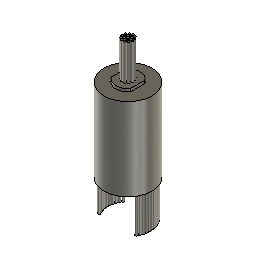
single_axis_test_jig (Autodesk Fusion 360 archive; units mm, degrees)
design "slip_ring_6.75Rx23.2Lmm"
Autodesk Fusion 360 part; units mm, degrees
note: some values were not read from the file. Set by a fixed rule: which sketch regions a step uses.
(part 1 of 4)
sketch "Sketch1" plane through (0, 0, 0) normal (0, 0, 1) x (1, 0, 0)
sketch "Sketch2" plane through (0, 0, 0) normal (0, 0, 1) x (1, 0, 0)
  circle A0 centre (0, 0) radius 6.75
  dimension "d1" = 13.5
  constraint coincident A0.centre origin
  measures "d1" diameter of A0
extrude "Extrude1" add sketch "Sketch2" along normal blind 23.2
sketch "Sketch3" plane through (0, 0, 23.2) normal (0, 0, 1) x (-1, 0, 0)
  circle A0 centre (0, 0) radius 6.75
  line L0 (-2.75, -1.9994) -> (-2.75, 1.9994)
  line L1 (2.75, 1.9994) -> (2.75, -1.9994)
  arc A1 (2.75, 1.9994) -> (-2.75, 1.9994) centre (0, 0) ccw
  arc A2 (-2.75, -1.9994) -> (2.75, -1.9994) centre (0, 0) ccw
  dimension "d4" = 6.8
  constraint coincident A0.centre A1.centre
  constraint vertical L0
  constraint vertical L1
  constraint concentric A1 A2
  measures "d4" diameter of A1
extrude "Extrude2" add sketch "Sketch3" along normal blind 0.8 contours L0 L1 A1 A2
sketch "Sketch5" plane through (0, 0, 24) normal (0, 0, 1) x (-1, 0, 0)
  arc A0 (2.75, 1.9994) -> (-2.75, 1.9994) centre (0, 0) ccw
  line L0 (-2.75, 1.9994) -> (-2.75, -1.9994)
  arc A1 (-2.75, -1.9994) -> (2.75, -1.9994) centre (0, 0) ccw
  line L1 (2.75, -1.9994) -> (2.75, 1.9994)
  circle A2 centre (0, 0) radius 0.3
  circle A3 centre (0, -0.7865) radius 0.3
  circle A4 centre (0.5561, -0.5561) radius 0.3
  circle A5 centre (0.7865, 0) radius 0.3
  circle A6 centre (0.5561, 0.5561) radius 0.3
  circle A7 centre (0, 0.7865) radius 0.3
  circle A8 centre (-0.5561, 0.5561) radius 0.3
  circle A9 centre (-0.7865, 0) radius 0.3
  circle A10 centre (-0.5561, -0.5561) radius 0.3
  circle A11 centre (0.007, -1.4) radius 0.3
  circle A12 centre (0.7628, -1.174) radius 0.3
  circle A13 centre (1.2764, -0.5752) radius 0.3
  circle A14 centre (1.3848, 0.2061) radius 0.3
  circle A15 centre (1.0535, 0.9221) radius 0.3
  circle A16 centre (0.3877, 1.3453) radius 0.3
  circle A17 centre (-0.4011, 1.3413) radius 0.3
  circle A18 centre (-1.0626, 0.9115) radius 0.3
  circle A19 centre (-1.3867, 0.1923) radius 0.3
  circle A20 centre (-1.2706, -0.5879) radius 0.3
  circle A21 centre (-0.751, -1.1815) radius 0.3
  dimension "d18" = 0.6
  dimension "d19" = 0.6
  dimension "d21" = 360
  dimension "d22" = 0.6
  dimension "d23" = 0.7865
  dimension "d24" = 1.4
  dimension "d26" = 360
  constraint coincident A0.centre A1.centre
  measures "d18" diameter of A2
  measures "d19" diameter of A3
  measures "d22" diameter of A11
  measures "d23" distance of A0.centre A3.centre
  measures "d24" vertical distance of A0.centre A11.centre
extrude "Extrude4" add sketch "Sketch5" along normal blind 10 contours A2 | A3 | A4 | A10 | A5 | A9 | A6 | A8 | A7 | A11 | A12 | A13 | A14 | A15 | A16 | A17 | A18 | A19 | A20 | A21
sketch "Sketch6" plane through (0, 0, 0) normal (0, 0, -1) x (1, 0, 0)
  circle A0 centre (0, 0) radius 6.75
  circle A1 centre (0, 0) radius 5.25
  circle A2 centre (0, 0) radius 6 construction
  circle A3 centre (-6, 0) radius 0.35
  circle A4 centre (-5.9527, -0.752) radius 0.35
  circle A5 centre (-5.8115, -1.4921) radius 0.35
  circle A6 centre (-5.5787, -2.2087) radius 0.35
  circle A7 centre (-5.2578, -2.8905) radius 0.35
  circle A8 centre (-4.8541, -3.5267) radius 0.35
  circle A9 centre (4.8541, -3.5267) radius 0.35
  circle A10 centre (5.2578, -2.8905) radius 0.35
  circle A11 centre (5.5787, -2.2087) radius 0.35
  circle A12 centre (5.8115, -1.4921) radius 0.35
  circle A13 centre (5.9527, -0.752) radius 0.35
  circle A14 centre (6, 0) radius 0.35
  circle A15 centre (5.9527, 0.752) radius 0.35
  circle A16 centre (5.8115, 1.4921) radius 0.35
  circle A17 centre (5.5787, 2.2087) radius 0.35
  circle A18 centre (5.2578, 2.8905) radius 0.35
  circle A19 centre (-5.2578, 2.8905) radius 0.35
  circle A20 centre (-5.5787, 2.2087) radius 0.35
  circle A21 centre (-5.8115, 1.4921) radius 0.35
  circle A22 centre (-5.9527, 0.752) radius 0.35
  dimension "d29" = 10.5
  dimension "d30" = 12
  dimension "d31" = 0.7
  dimension "d33" = 360
  constraint concentric A0 A1
  constraint concentric A1 A2
  constraint coincident A2 A3.centre
  measures "d29" diameter of A1
  measures "d30" diameter of A2
  measures "d31" diameter of A3
extrude "Extrude5" add sketch "Sketch6" along normal blind 10 contours A3 | A4 | A5 | A6 | A7 | A8 | A9 | A10 | A11 | A12 | A13 | A14 | A15 | A16 | A17 | A18 | A19 | A20 | A21 | A22

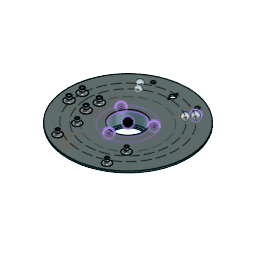
design "top_plate"
Autodesk Fusion 360 part; units mm, degrees
sketch "Sketch1" plane through (0, 0, 0) normal (0, 0, 1) x (1, 0, 0)
  circle A0 centre (0, 0) radius 80
  dimension "d1" = 160
  constraint coincident A0.centre origin
  measures "d1" diameter of A0
extrude "Extrude1" add sketch "Sketch1" along normal blind 2
sketch "Sketch4" plane through (0, 0, 2) normal (0, 0, 1) x (-1, 0, 0)
  circle A0 centre (0, 0) radius 80
  circle A1 centre (0, 0) radius 18
  dimension "d9" = 36
  constraint concentric A0 A1
  measures "d9" diameter of A1
extrude "Extrude3" cut sketch "Sketch4" against normal blind 20 contours A1
sketch "Sketch5" plane through (0, 0, 2) normal (0, 0, 1) x (-1, 0, 0)
  circle A0 centre (0, 0) radius 18
  circle A1 centre (0, 0) radius 80
  circle A2 centre (0, 0) radius 21
  circle A3 centre (0, 0) radius 30
  dimension "d12" = 42
  dimension "d13" = 60
  constraint coincident A0.centre A1.centre
  constraint concentric A2 A3
  measures "d12" diameter of A2
  measures "d13" diameter of A3
extrude "Extrude4" add sketch "Sketch5" against normal blind 19 contours A3
sketch "Sketch6" plane through (0, 0, 2) normal (0, 0, -1) x (-1, 0, 0)
  circle A0 centre (0, 0) radius 21
  circle A1 centre (0, 0) radius 28
  circle A2 centre (0, -25.5) radius 1.6
  circle A3 centre (0, 0) radius 80
  circle A4 centre (0, 0) radius 18
  dimension "d118" = 3.2
  dimension "d119" = 25.5
  constraint vertical A0.centre A2.centre
  measures "d118" diameter of A2
  measures "d119" distance of A0.centre A2.centre
extrude "Extrude5" cut sketch "Sketch6" along normal blind 6.3 contours A2
pattern_circular "C-Pattern2" count 3 over 360 about axis through (0, 0, 2) along (0, 0, -1) of "Extrude5"
sketch "Sketch7" plane through (0, 0, 0) normal (0, 0, -1) x (1, 0, 0)
  circle A0 centre (0, 0) radius 18
  circle A1 centre (0, 0) radius 80
  circle A2 centre (0, 0) radius 45 construction
  circle A3 centre (0, 0) radius 21
  circle A4 centre (0, 0) radius 30
  dimension "d21" = 90
  constraint concentric A0 A2
  measures "d21" diameter of A2
sketch "Sketch8" plane through (0, 0, 0) normal (0, 0, -1) x (1, 0, 0)
  circle A0 centre (0, -60) radius 3.5
  circle A1 centre (0, -65.5) radius 1
  circle A2 centre (0, -54.5) radius 1
  dimension "d22" = 7
  dimension "d23" = 2
  dimension "d24" = 2
  measures "d22" diameter of A0
  measures "d23" diameter of A1
  measures "d24" diameter of A2
extrude "Extrude6" cut sketch "Sketch8" against normal blind 2
move_face "OffsetFaces1" offset -0.2 1 faces at (20.8956, -2.0909, -11.3333)
ref_plane "WorkPlane1" through (0, 0, 12.125) normal (-0.819152, 0.573576, 0) x (0, 0, 1)
ref_plane "WorkPlane2" through (0, 0, 12.125) normal (-0.819152, -0.573576, 0) x (0, 0, 1)
sketch "Sketch9" plane through (0, 0, 2) normal (0, 0, 1) x (-1, 0, 0)
  circle A0 centre (0, 0) radius 80
  circle A1 centre (0, 0) radius 55 construction
  circle A2 centre (0, 0) radius 64.5 construction
  circle A3 centre (-22.0836, -12.75) radius 1.6
  circle A4 centre (22.0836, -12.75) radius 1.6
  circle A5 centre (0, 25.5) radius 1.6
  dimension "d31" = 110
  dimension "d32" = 129
  constraint coincident A0.centre A1.centre
  constraint concentric A0 A2
  measures "d31" diameter of A1
  measures "d32" diameter of A2
sketch "Sketch10" plane through (0, 0, 0) normal (-0.819152, -0.573576, 0) x (0, 0, 1)
  line L0 (2, 55) -> (2, 64.5) construction
  line L1 (2, 64.5) -> (2, 65)
  dimension "d34" = 9.5
  dimension "d43" = 0.5
  constraint vertical L0
  constraint parallel L0 L1
  measures "d34" distance of L0.start L0.end
  measures "d43" distance of L0.end L1.end
sketch "Sketch11" plane through (0, 0, 0) normal (-0.819152, 0.573576, 0) x (0, 0, 1)
  line L0 (2, 55) -> (2, 64.5) construction
  line L1 (2, 64.5) -> (2, 65) construction
  dimension "d36" = 9.5
  constraint vertical L0
  constraint parallel L0 L1
  measures "d36" distance of L0.start L0.end
sketch "Sketch12" plane through (0, 0, 2) normal (0, 0, 1) x (-1, 0, 0)
  circle A0 centre (-36.9957, -52.8353) radius 1.25
  circle A1 centre (-31.5467, -45.0534) radius 1.25
  circle A2 centre (31.5467, -45.0534) radius 1.25
  circle A3 centre (36.9957, -52.8353) radius 1.25
  point P0 (-36.9957, -52.8353)
  point P1 (-31.5467, -45.0534)
  point P2 (31.5467, -45.0534)
  point P3 (36.9957, -52.8353)
  dimension "d37" = 2.5
  dimension "d38" = 2.5
  dimension "d39" = 2.5
  dimension "d40" = 2.5
  constraint coincident P0 A0.centre
  constraint coincident P1 A1.centre
  constraint coincident P2 A2.centre
  constraint coincident P3 A3.centre
  measures "d37" diameter of A0
  measures "d38" diameter of A1
  measures "d39" diameter of A2
  measures "d40" diameter of A3
extrude "Extrude7" cut sketch "Sketch12" against normal blind 2
sketch "Sketch13" plane through (0, 0, 2) normal (0, 0, 1) x (-1, 0, 0)
  circle A0 centre (37.2825, -53.2449) radius 1.25
  point P0 (37.2825, -53.2449)
  dimension "d44" = 2.5
  constraint coincident P0 A0.centre
  measures "d44" diameter of A0
sketch "Sketch14" plane through (0, 0, 2) normal (0, 0, 1) x (-1, 0, 0)
  point P0 (-37.2825, -53.2449)
sketch "Sketch15" plane through (0, 0, 2) normal (0, 0, 1) x (-1, 0, 0)
  line L0 (-38.0196, -52.1183) -> (-38.3064, -52.5279)
  circle A0 centre (-37.2825, -53.2449) radius 1.25
  circle A1 centre (-36.9957, -52.8353) radius 1.25
  line L1 (-35.9717, -53.5523) -> (-36.2585, -53.9619)
  circle A2 centre (-31.5467, -45.0534) radius 1.25
  circle A3 centre (31.5467, -45.0534) radius 1.25
  circle A4 centre (-36.9957, -52.8353) radius 1.25
  circle A5 centre (36.9957, -52.8353) radius 1.25
  circle A6 centre (0, -60) radius 3.5
  circle A7 centre (0, -65.5) radius 1
  circle A8 centre (0, -54.5) radius 1
  circle A9 centre (0, 0) radius 80
  circle A10 centre (0, 0) radius 18
  circle A11 centre (-22.0836, -12.75) radius 1.6
  circle A12 centre (22.0836, -12.75) radius 1.6
  circle A13 centre (0, 25.5) radius 1.6
  point P0 (-36.9957, -52.8353)
  constraint tangent L0 A0
  constraint coincident L0.end A0
  constraint coincident L0.start A1
  constraint tangent A1 L1
  constraint coincident A1 L1.start
  constraint coincident A0 L1.end
  constraint coincident P0 A1.centre
extrude "Extrude8" cut sketch "Sketch15" against normal blind 2 contours L0 A0 A1 A4 | A0 A1 A4 | A0 A1 L1 A4 picked at (-38.0226, -54.0336)
sketch "Sketch16" plane through (0, 0, 2) normal (0, 0, 1) x (-1, 0, 0)
  line L0 (36.2585, -53.9619) -> (35.9717, -53.5523)
  line L1 (31.5467, -45.0534) -> (36.9957, -52.8353)
  circle A0 centre (37.2825, -53.2449) radius 1.25
  circle A1 centre (36.9957, -52.8353) radius 1.25
  line L2 (38.3064, -52.5279) -> (38.0196, -52.1183)
  constraint parallel L0 L1
  constraint tangent L0 A0
  constraint coincident L0.start A0
  constraint coincident L0.end A1
  constraint parallel L1 L2
  constraint tangent A1 L2
  constraint coincident A1 L2.end
  constraint coincident A0 L2.start
extrude "Extrude9" cut sketch "Sketch16" sketch "Sketch13" against normal blind 2 contours L0 A0 A1 | A0 A1 L2 of sketch 2
move_face "OffsetFaces3" offset 0.4 1 faces at (21.0947, -2.1108, -5.6667)
move_face "OffsetFaces4" offset -0.3 1 faces at (4.8751, -17.3272, 0.6667)
move_face "OffsetFaces5" offset -0.2 1 faces at (3.4826, 60.3485, 0.6667)
move_face "OffsetFaces8" offset -0.15 10 faces at (-32.6985, 44.5678, 0.6667) (-37.0808, 54.4785, 0.6667) (-36.0673, 53.6888, 0.6667) (-35.9054, 53.4468, 0.6667) (-38.1152, 52.2549, 0.6667) (32.2249, 46.1034, 0.6667) (37.9826, 52.0682, 0.6667) (36.1629, 53.8253, 0.6667) (38.3727, 52.6334, 0.6667) (38.2108, 52.3914, 0.6667)
move_face "OffsetFaces9" offset -0.15 2 faces at (-0.9215, 54.8884, 1.3333) (-0.9802, 65.3019, 1.3333)
sketch "Sketch17" plane through (0, 0, 2) normal (0, 0, 1) x (-1, 0, 0)
  line L0 (0, 35) -> (0, 61.15) construction
  line L1 (0, 35) -> (-33.075, 35) construction
  line L2 (0, 35) -> (33.075, 35) construction
  line L3 (0, 61.15) -> (-33.075, 61.15) construction
  line L4 (0, 61.15) -> (33.075, 61.15) construction
  circle A0 centre (33.075, 35) radius 2.5
  circle A1 centre (-33.075, 35) radius 2.5
  circle A2 centre (33.075, 61.15) radius 2.5
  circle A3 centre (-33.075, 61.15) radius 2.5
  dimension "d59" = 26.15
  dimension "d60" = 33.075
  dimension "d61" = 33.075
  dimension "d62" = 33.075
  dimension "d63" = 33.075
  dimension "d64" = 5
  dimension "d65" = 5
  dimension "d66" = 5
  dimension "d67" = 5
  constraint vertical L0
  constraint perpendicular L0 L1
  constraint perpendicular L0 L2
  constraint perpendicular L0 L3
  constraint perpendicular L0 L4
  constraint coincident L2.end A0.centre
  constraint coincident L1.end A1.centre
  constraint coincident L4.end A2.centre
  constraint coincident L3.end A3.centre
  measures "d59" distance of L0.start L0.end
  measures "d60" distance of L0.start L1.end
  measures "d61" distance of L0.start L2.end
  measures "d62" distance of L0.end L3.end
  measures "d63" distance of L0.end L4.end
  measures "d64" diameter of A0
  measures "d65" diameter of A1
  measures "d66" diameter of A2
  measures "d67" diameter of A3
extrude "Extrude11" add sketch "Sketch17" along normal blind 6
fillet "Fillet1" radius 3 4 edges at (-30.7442, -62.054, 2) (-30.7442, -35.904, 2) (35.4058, -35.904, 2) (35.4058, -62.054, 2)
sketch "Sketch18" plane through (0, 0, 8) normal (0, 0, 1) x (-1, 0, 0)
  circle A0 centre (33.075, 35) radius 2.5
  circle A1 centre (33.075, 35) radius 1.55
  dimension "d73" = 3.1
  constraint concentric A0 A1
  measures "d73" diameter of A1
sketch "Sketch19" plane through (0, 0, 8) normal (0, 0, 1) x (-1, 0, 0)
  circle A0 centre (33.075, 61.15) radius 2.5
  circle A1 centre (33.075, 61.15) radius 1.55
  dimension "d74" = 3.1
  constraint concentric A0 A1
  measures "d74" diameter of A1
sketch "Sketch20" plane through (0, 0, 8) normal (0, 0, 1) x (-1, 0, 0)
  circle A0 centre (-33.075, 61.15) radius 2.5
  circle A1 centre (-33.075, 61.15) radius 1.55
  dimension "d75" = 3.1
  constraint concentric A0 A1
  measures "d75" diameter of A1
sketch "Sketch21" plane through (0, 0, 8) normal (0, 0, 1) x (-1, 0, 0)
  circle A0 centre (-33.075, 35) radius 2.5
  circle A1 centre (-33.075, 35) radius 1.55
  dimension "d76" = 3.1
  constraint concentric A0 A1
  measures "d76" diameter of A1
extrude "Extrude12" cut sketch "Sketch20" sketch "Sketch19" sketch "Sketch18" sketch "Sketch21" against normal blind 5 contours A1 of sketch 2 contours A1 of sketch 3 contours A1 of sketch 4 contours A1
sketch "Sketch22" plane through (0, 0, 2) normal (0, 0, 1) x (-1, 0, 0)
  line L0 (42, 0) -> (64.86, 0) construction
  line L1 (42, 0) -> (42, 14.113) construction
  line L2 (64.86, 0) -> (64.86, 14.113) construction
  line L3 (42, 0) -> (42, -3.667) construction
  line L4 (64.86, 0) -> (64.86, -3.667) construction
  circle A0 centre (64.86, -3.667) radius 3
  circle A1 centre (64.86, 14.113) radius 3
  circle A2 centre (42, -3.667) radius 3
  circle A3 centre (42, 14.113) radius 3
  dimension "d79" = 22.86
  dimension "d80" = 14.113
  dimension "d81" = 14.113
  dimension "d82" = 3.667
  dimension "d83" = 3.667
  dimension "d84" = 6
  dimension "d85" = 6
  dimension "d86" = 6
  dimension "d87" = 6
  constraint horizontal L0
  constraint perpendicular L0 L1
  constraint perpendicular L0 L2
  constraint perpendicular L0 L3
  constraint perpendicular L0 L4
  constraint coincident L4.end A0.centre
  constraint coincident L2.end A1.centre
  constraint coincident L3.end A2.centre
  constraint coincident L1.end A3.centre
  measures "d79" distance of L0.start L0.end
  measures "d80" distance of L0.start L1.end
  measures "d81" distance of L0.end L2.end
  measures "d82" distance of L0.start L3.end
  measures "d83" distance of L0.end L4.end
  measures "d84" diameter of A0
  measures "d85" diameter of A1
  measures "d86" diameter of A2
  measures "d87" diameter of A3
extrude "Extrude13" add sketch "Sketch22" along normal blind 6
fillet "Fillet2" radius 3 4 edges at (-62.063, -15.1978, 2) (-39.203, -15.1978, 2) (-39.203, 2.5822, 2) (-62.063, 2.5822, 2)
sketch "Sketch23" plane through (0, 0, 8) normal (0, 0, 1) x (-1, 0, 0)
  circle A0 centre (42, -3.667) radius 3
  circle A1 centre (42, -3.667) radius 2.2
  dimension "d92" = 4.4
  constraint concentric A0 A1
  measures "d92" diameter of A1
sketch "Sketch24" plane through (0, 0, 8) normal (0, 0, 1) x (-1, 0, 0)
  circle A0 centre (42, 14.113) radius 3
  circle A1 centre (42, 14.113) radius 2.2
  dimension "d93" = 4.4
  constraint concentric A0 A1
  measures "d93" diameter of A1
sketch "Sketch25" plane through (0, 0, 8) normal (0, 0, 1) x (-1, 0, 0)
  circle A0 centre (64.86, 14.113) radius 3
  circle A1 centre (64.86, 14.113) radius 2.2
  dimension "d94" = 4.4
  constraint concentric A0 A1
  measures "d94" diameter of A1
sketch "Sketch26" plane through (0, 0, 8) normal (0, 0, 1) x (-1, 0, 0)
  circle A0 centre (64.86, -3.667) radius 3
  circle A1 centre (64.86, -3.667) radius 2.2
  dimension "d95" = 4.4
  constraint concentric A0 A1
  measures "d95" diameter of A1
extrude "Extrude14" cut sketch "Sketch26" sketch "Sketch25" sketch "Sketch24" sketch "Sketch23" against normal blind 5 contours A1 of sketch 2 contours A1 of sketch 3 contours A1 of sketch 4 contours A1
sketch "Sketch27" plane through (0, 0, -17) normal (0, 0, -1) x (1, 0, 0)
  circle A0 centre (0, 0) radius 20.8
  circle A1 centre (0, 0) radius 30
  circle A2 centre (0, -24.5) radius 2.2
  circle A3 centre (-21.2176, 12.25) radius 2.2
  circle A4 centre (21.2176, 12.25) radius 2.2
sketch "Sketch28" plane through (0, 0, -17) normal (0, 0, -1) x (1, 0, 0)
  circle A0 centre (0, 0) radius 20.8
  circle A1 centre (0, 0) radius 30
  circle A2 centre (-0.3894, 0) radius 18
  dimension "d103" = 36
  measures "d103" diameter of A2
extrude "Extrude16" add sketch "Sketch28" against normal blind 2 contours A0
sketch "Sketch29" plane through (0, 0, 2) normal (0, 0, 1) x (-1, 0, 0)
sketch "Sketch30" plane through (0, 0, 2) normal (0, 0, 1) x (-1, 0, 0)
  circle A0 centre (0, 0) radius 21.075
  dimension "d106" = 42.15
  constraint coincident A0.centre origin
  measures "d106" diameter of A0
extrude "Extrude17" cut sketch "Sketch30" against normal blind 17
sketch "Sketch31" plane through (0, 0, 2) normal (0, 0, 1) x (-1, 0, 0)
  circle A0 centre (0, 0) radius 70 construction
  circle A1 centre (29.7262, -63.3747) radius 2.6
  circle A2 centre (-29.7262, -63.3747) radius 2.6
  line L0 (31.5467, -45.0534) -> (36.9957, -52.8353)
  line L1 (-31.5467, -45.0534) -> (-36.9957, -52.8353)
  dimension "d109" = 5.2
  dimension "d110" = 5.2
  dimension "d111" = 12
  dimension "d112" = 12
  dimension "d115" = 140
  constraint coincident A0.centre origin
  constraint coincident A0 A1.centre
  constraint coincident A0 A2.centre
  measures "d109" diameter of A1
  measures "d110" diameter of A2
  measures "d111" distance of A1.centre L0
  measures "d112" distance of A2.centre L1
  measures "d115" diameter of A0
extrude "Extrude18" cut sketch "Sketch31" against normal blind 3
sketch "Sketch32" plane through (0, 0, -17) normal (0, 0, -1) x (1, 0, 0)
  circle A0 centre (0, 0) radius 30
  circle A1 centre (0, 0) radius 18
  circle A2 centre (-0.3894, 0) radius 18
  dimension "d120" = 36
  measures "d120" diameter of A1
chamfer "Chamfer1" distance 0.2 angle 45 4 edges at (34.5201, -35.5605, 8) (34.5201, -61.7105, 8) (-31.6299, -61.7105, 8) (-31.6299, -35.5605, 8)
chamfer "Chamfer1" distance 0.2 angle 45 4 edges at (-39.9489, -14.9086, 8) (-39.9489, 2.8714, 8) (-62.8089, 2.8714, 8) (-62.8089, -14.9086, 8)
equation "d119 = ( 51 / 2 ) * 1 mm"

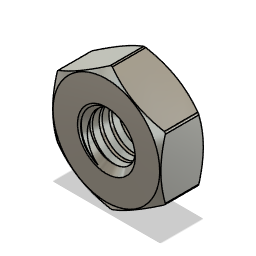
design "M2.5x2mm_hex_nut"
Autodesk Fusion 360 part; units mm, degrees
sketch "Skizze1" plane through (0, 0, 0) normal (0, 0, 1) x (1, 0, 0)
  line L0 (-2.5, -1.4434) -> (0, -2.8868)
  line L1 (0, -2.8868) -> (2.5, -1.4434)
  line L2 (2.5, -1.4434) -> (2.5, 1.4434)
  line L3 (2.5, 1.4434) -> (0, 2.8868)
  line L4 (0, 2.8868) -> (-2.5, 1.4434)
  line L5 (-2.5, 1.4434) -> (-2.5, -1.4434)
  dimension "d3" = 2.5
  constraint vertical L5
  measures "d3" distance of origin L5
extrude "Extrusion1" add sketch "Skizze1" along normal mid plane 2
sketch "Skizze2" plane through (0, 0, 1) normal (0, 0, 1) x (1, 0, 0)
  line L0 (-2.5, 1.4434) -> (-2.5, -1.4434)
  line L1 (-2.5, -1.4434) -> (0, -2.8868)
  line L2 (0, -2.8868) -> (2.5, -1.4434)
  line L3 (2.5, -1.4434) -> (2.5, 1.4434)
  line L4 (2.5, 1.4434) -> (0, 2.8868)
  line L5 (0, 2.8868) -> (-2.5, 1.4434)
hole "Bohrung1" at (0, 0, 1) direction (0, 0, -1) diameter 2.076 end through all
thread "Gewinde1" "ISO Metric profile 2.5 M2.5x0.45 6H" major diameter 2.58 minor diameter 2.0755 pitch 0.45 angle 60 modelled right hand crest width 0.1211 on face at (0.1034, -1.0328, -0.3333) crest through (1.0377, 0, 0.8875)
sketch "Skizze4" plane through (0, 0, 0) normal (1, 0, 0) x (0, 0, -1)
  line L0 (1, 1.4434) -> (1, 2.8868)
  line L1 (1, -2.8868) -> (1, -1.4434)
  line L2 (1, 2.8868) -> (-1, 2.8868)
  line L3 (0.7575, 2.8868) -> (1, 2.4668)
  line L4 (1, 2.8868) -> (0.8181, 2.7818) construction
  line L5 (1, 2.4668) -> (1, 0)
  line L6 (0.7575, 2.8868) -> (0, 2.8868)
  line L7 (0, 1.75) -> (0, 22.5) construction
  line L8 (-0.7575, 2.8868) -> (0, 2.8868)
  line L9 (-0.7575, 2.8868) -> (-1, 2.4668)
  line L10 (-1, 2.4668) -> (-1, 0)
  line L11 (-1, 0) -> (1, 0)
  line L12 (-1, 3.3068) -> (0, 3.3068)
  line L13 (1, 3.3068) -> (0, 3.3068)
  line L14 (1, 3.3068) -> (1.42, 2.5793)
  line L15 (1.42, 2.5793) -> (1.42, -0.42)
  line L16 (-1.42, -0.42) -> (1.42, -0.42)
  line L17 (-1.42, 2.5793) -> (-1.42, -0.42)
  line L18 (-1, 3.3068) -> (-1.42, 2.5793)
  line L19 (-1, 0) -> (-1.42, 0)
  line L20 (1, 0) -> (1.42, 0)
  line L21 (1, -1.4434) -> (1, 1.4434)
  line L22 (-1.75, 0) -> (-22.5, 0)
  dimension "d18" = 0.21
  dimension "d19" = 0.42
  dimension "d23" = 150
  constraint coincident L2 L3.start
  constraint coincident L0 L3.end
  constraint coincident L0.end L2.start
  constraint midpoint L2 L6.end
  constraint symmetric L3.start L7 L8.start
  constraint symmetric L3.end L7 L9.end
  constraint symmetric L5.end L7 L10.end
  constraint symmetric L6.end L7 L8.end
  constraint coincident L17 L19.end
  constraint perpendicular L17 L19
  constraint coincident L15 L20.end
  constraint perpendicular L15 L20
  constraint perpendicular L3 L4
  constraint coincident L3 L4.end
  constraint vertical L10
  constraint collinear L19 L22
  measures "d18" distance of L0.end L4.end
  measures "d23" angle of L3 L5
revolve "Drehen1" cut sketch "Skizze4" angle 360 about axis through (0, 0, 1.75) along (0, 0, 1) contours L0 L2 L5 L6 L8 L9 L10 L12 L13 L14 L15 L17 L18 L19 L20 L21 | L0 L2 L3
fillet "Abrundung1" radius 0.1 6 edges at (2.5, 1.4434, 0) (2.5, -1.4434, 0) (0, -2.8868, 0) (-2.5, -1.4434, 0) (0, 2.8868, 0) (-2.5, 1.4434, 0)
sketch "Skizze5" plane through (0, 0, 0) normal (1, 0, 0) x (0, 0, -1)
  line L0 (-1, 1.3328) -> (-0.7172, 1.05)
  line L1 (-0.7172, 1.05) -> (0, 1.05)
  line L2 (0, 1.75) -> (0, 22.5)
  line L3 (0, 1.05) -> (0, 0) construction
  line L4 (-0.7172, 1.05) -> (-1, 1.05) construction
  line L5 (-1, 1.05) -> (-0.8586, 1.1914) construction
  line L6 (-1, 1.3328) -> (-1, 0)
  line L7 (-1, 0) -> (0, 0)
  line L8 (0.7172, 1.05) -> (0, 1.05)
  line L9 (1, 1.3328) -> (0.7172, 1.05)
  line L10 (1, 1.3328) -> (1, 0)
  line L11 (1, 0) -> (0, 0)
  line L12 (-1, 2.4668) -> (-1, -2.4668)
  dimension "d28" = 1.05
  dimension "d29" = 0.2
  dimension "d31" = 45
  constraint horizontal L1
  constraint coincident L1.end L2
  constraint coincident L3.end L7.end
  constraint coincident L0 L5.end
  constraint perpendicular L0 L5
  constraint symmetric L0.start L2 L9.start
  constraint symmetric L0.end L2 L8.start
  constraint symmetric L1.end L2 L3.start
  constraint symmetric L2 L6.end L10.end
  constraint symmetric L2 L3.end L7.end
  constraint horizontal L7
  constraint vertical L6
  constraint horizontal L4
  constraint coincident L4.end L6
  constraint collinear L6 L12
  measures "d28" distance of L1.end L3.end
  measures "d29" distance of L4.end L5.end
  measures "d31" angle of L0 L6
revolve "Drehen2" cut sketch "Skizze5" angle 360 about axis through (0, 0, 1.75) along (0, 0, 1)
equation "HexWidth = 5 mm" comment "Side-to-side width"
equation "Height = 2 mm"
equation "d3 = HexWidth / 2"
equation "d4 = Height"
equation "ChamferDepth = 0.21 mm" comment "Corner chamfer depth"
equation "ChamferAngle = 30 deg" comment "Corner chamfer angle"
equation "ThreadChamferDepth = 0.2 mm"
equation "d18 = ChamferDepth"
equation "d19 = 2 * ChamferDepth"
equation "SideFillet = 0.1 mm" comment "Fillet of the sides"
equation "d22 = SideFillet"
equation "d23 = 180 deg - ChamferAngle"
equation "ThreadChamferAngle = 45 deg"
equation "CoreDrill = 2.1 mm" comment "Core drill size for the given thread. Used to compute the thread chamfer."
equation "d28 = CoreDrill / 2"
equation "d29 = ThreadChamferDepth"
equation "d31 = ThreadChamferAngle"
named bodies: "Nut"

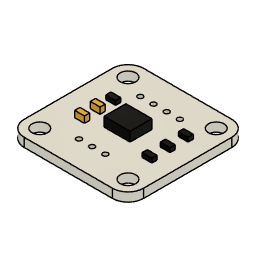
design "AS5600"
Autodesk Fusion 360 part; units mm, degrees
sketch "Sketch2" plane through (0, 0, 0) normal (0, 1, 0) x (1, 0, 0)
  line L0 (-8.5, -11.5) -> (8.5, -11.5)
  line L1 (11.5, -8.5) -> (11.5, 8.5)
  line L2 (8.5, 11.5) -> (-8.5, 11.5)
  line L3 (-11.5, 8.5) -> (-11.5, -8.5)
  line L4 (-11.5, -11.5) -> (11.5, 11.5) construction
  line L5 (11.5, -11.5) -> (-11.5, 11.5) construction
  line L6 (-8.5, 8.5) -> (8.5, 8.5) construction
  line L7 (8.5, 8.5) -> (8.5, -8.5) construction
  line L8 (8.5, -8.5) -> (-8.5, -8.5) construction
  line L9 (-8.5, -8.5) -> (-8.5, 8.5) construction
  line L10 (-8.5, 8.5) -> (8.5, -8.5) construction
  line L11 (8.5, 8.5) -> (-8.5, -8.5) construction
  circle A0 centre (-8.5, 8.5) radius 1.5
  circle A1 centre (8.5, 8.5) radius 1.5
  circle A2 centre (8.5, -8.5) radius 1.5
  circle A3 centre (-8.5, -8.5) radius 1.5
  arc A4 (-8.5, 11.5) -> (-11.5, 8.5) centre (-8.5, 8.5) ccw
  arc A5 (11.5, 8.5) -> (8.5, 11.5) centre (8.5, 8.5) ccw
  arc A6 (8.5, -11.5) -> (11.5, -8.5) centre (8.5, -8.5) ccw
  arc A7 (-11.5, -8.5) -> (-8.5, -11.5) centre (-8.5, -8.5) ccw
  line L12 (-2.5, -2.1) -> (2.5, -2.1)
  line L13 (2.5, -2.1) -> (2.5, 2.1)
  line L14 (2.5, 2.1) -> (-2.5, 2.1)
  line L15 (-2.5, 2.1) -> (-2.5, -2.1)
  line L16 (-2.5, -2.1) -> (2.5, 2.1) construction
  line L17 (2.5, -2.1) -> (-2.5, 2.1) construction
  circle A8 centre (-4.12, 6.5) radius 0.5
  circle A9 centre (-1.58, 6.5) radius 0.5
  circle A10 centre (0.96, 6.5) radius 0.5
  circle A11 centre (3.5, 6.5) radius 0.5
  line L18 (-4.12, 6.5) -> (-1.58, 6.5) construction
  line L19 (-1.58, 6.5) -> (0.96, 6.5) construction
  line L20 (0.96, 6.5) -> (3.5, 6.5) construction
  circle A12 centre (2.14, -6.5) radius 0.5
  circle A13 centre (-0.4, -6.5) radius 0.5
  circle A14 centre (-2.94, -6.5) radius 0.5
  line L21 (-2.94, -6.5) -> (-0.4, -6.5) construction
  line L22 (-0.4, -6.5) -> (2.14, -6.5) construction
  line L23 (-6.9, 3.63) -> (-5.02, 3.63)
  line L24 (-5.02, 3.63) -> (-5.02, 2.63)
  line L25 (-5.02, 2.63) -> (-6.9, 2.63)
  line L26 (-6.9, 2.63) -> (-6.9, 3.63)
  line L27 (-6.9, 0.63) -> (-5.02, 0.63)
  line L28 (-5.02, 0.63) -> (-5.02, -0.37)
  line L29 (-5.02, -0.37) -> (-6.9, -0.37)
  line L30 (-6.9, -0.37) -> (-6.9, 0.63)
  line L31 (-6.9, -2.37) -> (-5.02, -2.37)
  line L32 (-5.02, -2.37) -> (-5.02, -3.37)
  line L33 (-5.02, -3.37) -> (-6.9, -3.37)
  line L34 (-6.9, -3.37) -> (-6.9, -2.37)
  line L35 (-6.9, 2.63) -> (-6.9, 0.63) construction
  line L36 (-6.9, -0.37) -> (-6.9, -2.37) construction
  line L37 (6.22, 4.5) -> (8.1, 4.5)
  line L38 (8.1, 4.5) -> (8.1, 3.5)
  line L39 (8.1, 3.5) -> (6.22, 3.5)
  line L40 (6.22, 3.5) -> (6.22, 4.5)
  line L41 (6.22, 1) -> (8.1, 1)
  line L42 (8.1, 1) -> (8.1, 0)
  line L43 (8.1, 0) -> (6.22, 0)
  line L44 (6.22, 0) -> (6.22, 1)
  line L45 (6.22, -2.5) -> (8.1, -2.5)
  line L46 (8.1, -2.5) -> (8.1, -3.5)
  line L47 (8.1, -3.5) -> (6.22, -3.5)
  line L48 (6.22, -3.5) -> (6.22, -2.5)
  line L49 (8.1, -2.5) -> (8.1, 0) construction
  line L50 (8.1, 3.5) -> (8.1, 1) construction
  dimension "d6" = 23
  dimension "d7" = 23
  dimension "d8" = 17
  dimension "d9" = 17
  dimension "d10" = 3
  dimension "d11" = 3
  dimension "d12" = 3
  dimension "d13" = 3
  dimension "d14" = 3
  dimension "d15" = 5
  dimension "d16" = 4.2
  dimension "d21" = 1
  dimension "d25" = 2.54
  dimension "d26" = 2.54
  dimension "d27" = 2.54
  dimension "d28" = 5
  dimension "d29" = 8
  dimension "d30" = 2.54
  dimension "d31" = 2.54
  dimension "d32" = 5
  dimension "d33" = 8.56
  dimension "d34" = 1.88
  dimension "d35" = 1
  dimension "d36" = 2
  dimension "d37" = 2
  dimension "d38" = 4.6
  dimension "d39" = 8.13
  dimension "d41" = 3.4
  dimension "d42" = 2.5
  dimension "d43" = 2.5
  dimension "d44" = 8
  constraint horizontal L0
  constraint perpendicular L0 L1
  constraint parallel L0 L2
  constraint parallel L1 L3
  constraint coincident L4 origin
  constraint coincident L5 origin
  constraint horizontal L6
  constraint perpendicular L6 L7
  constraint parallel L6 L8
  constraint parallel L7 L9
  constraint coincident L10 origin
  constraint coincident L11 origin
  constraint coincident L6.start L9.end
  constraint coincident L6.end L7.start
  constraint coincident L7.end L8.start
  constraint coincident L8.end L9.start
  constraint equal A0 A3
  constraint equal A1 A3
  constraint equal A2 A3
  constraint coincident L5.end L3
  constraint coincident L5.end L2
  constraint tangent L3 A4
  constraint tangent L2 A4
  constraint coincident L4.end L2
  constraint coincident L4.end L1
  constraint tangent L2 A5
  constraint tangent L1 A5
  constraint coincident L5.start L0
  constraint coincident L5.start L1
  constraint tangent L0 A6
  constraint tangent L1 A6
  constraint coincident L4.start L3
  constraint coincident L4.start L0
  constraint tangent L3 A7
  constraint tangent L0 A7
  constraint horizontal L12
  constraint perpendicular L12 L13
  constraint parallel L12 L14
  constraint parallel L13 L15
  constraint coincident L16 origin
  constraint coincident L17 origin
  constraint coincident A8.centre L18.start
  constraint coincident A9.centre L18.end
  constraint parallel L6 L18
  constraint coincident A10.centre L19.end
  constraint coincident A11.centre L20.end
  constraint horizontal L19
  constraint horizontal L20
  constraint equal A8 A9
  constraint equal A8 A10
  constraint equal A8 A11
  constraint equal A8 A14
  constraint equal A9 A13
  constraint equal A10 A12
  constraint coincident A14.centre L21.start
  constraint coincident A13.centre L21.end
  constraint horizontal L21
  constraint coincident A12.centre L22.end
  constraint horizontal L22
  constraint horizontal L23
  constraint vertical L24
  constraint horizontal L25
  constraint vertical L26
  constraint horizontal L27
  constraint vertical L28
  constraint horizontal L29
  constraint vertical L30
  constraint horizontal L31
  constraint vertical L32
  constraint horizontal L33
  constraint vertical L34
  constraint equal L23 L27
  constraint equal L27 L31
  constraint equal L24 L28
  constraint equal L28 L32
  constraint vertical L35
  constraint vertical L36
  constraint horizontal L37
  constraint vertical L38
  constraint horizontal L39
  constraint vertical L40
  constraint horizontal L41
  constraint vertical L42
  constraint horizontal L43
  constraint vertical L44
  constraint horizontal L45
  constraint vertical L46
  constraint horizontal L47
  constraint vertical L48
  constraint equal L23 L37
  constraint equal L24 L38
  constraint equal L23 L41
  constraint equal L24 L42
  constraint equal L23 L45
  constraint equal L24 L48
  constraint vertical L50
  constraint vertical L49
  measures "d6" distance of L4.start L5.start
  measures "d7" distance of L5.start L4.end
  measures "d8" distance of L7.end L8.end
  measures "d9" distance of L6.end L7.end
  measures "d10" diameter of A3
  measures "d11" radius of A4
  measures "d12" radius of A5
  measures "d13" radius of A6
  measures "d14" radius of A7
  measures "d15" distance of L13.end L14.end
  measures "d16" distance of L12.end L13.end
  measures "d21" diameter of A8
  measures "d25" distance of A8.centre A9.centre
  measures "d26" horizontal distance of A9.centre A10.centre
  measures "d27" horizontal distance of A10.centre A11.centre
  measures "d28" distance of L2 L18
  measures "d29" distance of L1 A11.centre
  measures "d30" distance of A13.centre A14.centre
  measures "d31" horizontal distance of A12.centre A13.centre
  measures "d32" distance of L0 L22
  measures "d33" distance of L3 A14.centre
  measures "d34" distance of L23.start L23.end
  measures "d35" distance of L23.end L24.end
  measures "d36" distance of L25 L27
  measures "d37" distance of L29 L31
  measures "d38" distance of L3 L35
  measures "d39" distance of L0 L33
  measures "d41" distance of L1 L50
  measures "d42" distance of L38.end L41.end
  measures "d43" distance of L42.end L45.end
  measures "d44" distance of L0 L47
extrude "Extrude1" add sketch "Sketch2" against normal blind 1.7 contours L0 L1 L2 L3 A4 A5 A6 A7 | L12 L13 L14 L15 | L23 L24 L25 L26 | L27 L28 L29 L30 | L31 L32 L33 L34 | L37 L38 L39 L40 | L41 L42 L43 L44 | L45 L46 L47 L48
extrude "Extrude2" add sketch "Sketch2" along normal blind 1.8 contours L12 L13 L14 L15
extrude "Extrude3" add sketch "Sketch2" along normal blind 0.8 contours L23 L24 L25 L26 | L37 L38 L39 L40 | L41 L42 L43 L44 | L45 L46 L47 L48
extrude "Extrude4" add sketch "Sketch2" along normal blind 1.22 contours L27 L28 L29 L30 | L31 L32 L33 L34

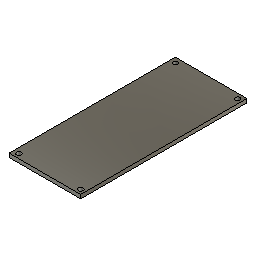
design "raspberry_pi_pico_mounting_board"
Autodesk Fusion 360 part; units mm, degrees
sketch "Sketch1" plane through (0, 0, 0) normal (0, 0, 1) x (1, 0, 0)
  line L0 (0, 0) -> (30.2, 0)
  line L1 (30.2, 0) -> (30.2, 70.15)
  line L2 (30.2, 70.15) -> (0, 70.15)
  line L3 (0, 70.15) -> (0, 0)
  dimension "d1" = 30.2
  dimension "d2" = 70.15
  constraint horizontal L0
  constraint vertical L1
  constraint horizontal L2
  constraint vertical L3
  constraint coincident L0.start L3.end
  measures "d1" distance of L0.start L0.end
  measures "d2" distance of L0.start L2.end
extrude "Extrude1" add sketch "Sketch1" along normal blind 1.6
sketch "Sketch3" plane through (0, 0, 1.6) normal (0, 0, 1) x (-1, 0, 0)
  line L0 (0, -70.15) -> (0, 0)
  line L1 (0, 0) -> (-30.2, 0)
  line L2 (-30.2, 0) -> (-30.2, -70.15)
  line L3 (-30.2, -70.15) -> (0, -70.15)
  circle A0 centre (-2.2, -68.05) radius 1
  circle A1 centre (-28.35, -68.05) radius 1
  circle A2 centre (-2.2, -1.9) radius 1
  circle A3 centre (-28.35, -1.9) radius 1
  dimension "d7" = 2
  dimension "d12" = -26.15
  dimension "d13" = 66.15
  measures "d7" diameter of A0
extrude "Extrude2" cut sketch "Sketch3" against normal blind 1.6 contours A0 | A1 | A2 | A3

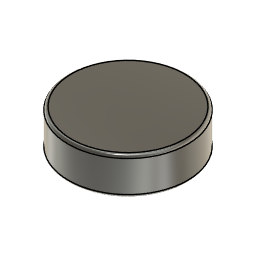
design "encoder_magnet"
Autodesk Fusion 360 part; units mm, degrees
sketch "Sketch1" plane through (0, 0, 0) normal (0, 0, 1) x (1, 0, 0)
  circle A0 centre (0, 0) radius 4
  dimension "d1" = 8
  constraint coincident A0.centre origin
  measures "d1" diameter of A0
extrude "Extrude1" add sketch "Sketch1" along normal blind 2.5
fillet "Fillet1" radius 0.2 1 edges at (-3.7293, -1.4465, 2.5)
fillet "Fillet2" radius 0.2 1 edges at (-3.7293, -1.4465, 0)

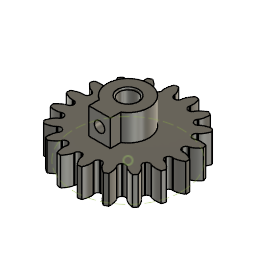
design "drive_gear"
description: Spur Gear; Module: 2.000000; Num Teeth: 18; Pressure Angle: 20.000000; Backlash: 0.00 mm
Autodesk Fusion 360 part; units mm, degrees
sketch "Sketch1" plane through (0, 0, 0) normal (0, 0, 1) x (1, 0, 0) in component "Spur Gear (18 teeth)"
  circle A0 centre (0, 0) radius 15.5492
extrude "Extrude1" add sketch "Sketch1" along normal blind 18 contours A0 picked at (5.718807, 1.412278) in component "Spur Gear (18 teeth)"
sketch "Sketch2" plane through (0, 0, 0) normal (0, 0, 1) x (1, 0, 0) in component "Spur Gear (18 teeth)"
  spline S0 degree 5 poles (16.82626, -1.72516) (16.835298, -1.72608) (16.853384, -1.727673) (16.880546, -1.72932) (16.916827, -1.730104) (16.962268, -1.729154) (17.007781, -1.726806) (17.053347, -1.723589) (17.098948, -1.719897) (17.144574, -1.715879) (17.19022, -1.711525) (17.235883, -1.706727) (17.281562, -1.701347) (17.327256, -1.695289) (17.372963, -1.688548) (17.418679, -1.681176) (17.464401, -1.673257) (17.510125, -1.664879) (17.555848, -1.656105) (17.601568, -1.646956) (17.647283, -1.637429) (17.692991, -1.627506) (17.738693, -1.617166) (17.784387, -1.606396) (17.83007, -1.595203) (17.875742, -1.583601) (17.9214, -1.57161) (17.967044, -1.559248) (18.012672, -1.546532) (18.058282, -1.533468) (18.103873, -1.520058) (18.149445, -1.506301) (18.194995, -1.492198) (18.240523, -1.47775) (18.286029, -1.46296) (18.331509, -1.447834) (18.376965, -1.432378) (18.422393, -1.416599) (18.467794, -1.400502) (18.513167, -1.38409) (18.558509, -1.367366) (18.603821, -1.350333) (18.649102, -1.332992) (18.694349, -1.315346) (18.739564, -1.297397) (18.784743, -1.279149) (18.829888, -1.260605) (18.874996, -1.241767) (18.920066, -1.222639) (18.965099, -1.203222) (19.010093, -1.18352) (19.055046, -1.163534) (19.099959, -1.143266) (19.144831, -1.122718) (19.18966, -1.101892) (19.234445, -1.08079) (19.279187, -1.059415) (19.323883, -1.037768) (19.368534, -1.015851) (19.413138, -0.993666) (19.457695, -0.971215) (19.502203, -0.948498) (19.546664, -0.925519) (19.591074, -0.902277) (19.635434, -0.878776) (19.679742, -0.855017) (19.723998, -0.831001) (19.768201, -0.806731) (19.812349, -0.782207) (19.856443, -0.75743) (19.900483, -0.732402) (19.935671, -0.712179) (19.962037, -0.696899) (19.979604, -0.686663) (19.988384, -0.681532) knots 0 0 0 0 0 0 0.01428571 0.02857143 0.04285714 0.05714286 0.07142857 0.08571429 0.1 0.11428571 0.12857143 0.14285714 0.15714286 0.17142857 0.18571429 0.2 0.21428571 0.22857143 0.24285714 0.25714286 0.27142857 0.28571429 0.3 0.31428571 0.32857143 0.34285714 0.35714286 0.37142857 0.38571429 0.4 0.41428571 0.42857143 0.44285714 0.45714286 0.47142857 0.48571429 0.5 0.51428571 0.52857143 0.54285714 0.55714286 0.57142857 0.58571429 0.6 0.61428571 0.62857143 0.64285714 0.65714286 0.67142857 0.68571429 0.7 0.71428571 0.72857143 0.74285714 0.75714286 0.77142857 0.78571429 0.8 0.81428571 0.82857143 0.84285714 0.85714286 0.87142857 0.88571429 0.9 0.91428571 0.92857143 0.94285714 0.95714286 0.97142857 0.98571429 1 1 1 1 1 1
  spline S1 degree 5 poles (16.82626, 1.72516) (16.835298, 1.72608) (16.853384, 1.727673) (16.880546, 1.72932) (16.916827, 1.730104) (16.962268, 1.729154) (17.007781, 1.726806) (17.053347, 1.723589) (17.098948, 1.719897) (17.144574, 1.715879) (17.19022, 1.711525) (17.235883, 1.706727) (17.281562, 1.701347) (17.327256, 1.695289) (17.372963, 1.688548) (17.418679, 1.681176) (17.464401, 1.673257) (17.510125, 1.664879) (17.555848, 1.656105) (17.601568, 1.646956) (17.647283, 1.637429) (17.692991, 1.627506) (17.738693, 1.617166) (17.784387, 1.606396) (17.83007, 1.595203) (17.875742, 1.583601) (17.9214, 1.57161) (17.967044, 1.559248) (18.012672, 1.546532) (18.058282, 1.533468) (18.103873, 1.520058) (18.149445, 1.506301) (18.194995, 1.492198) (18.240523, 1.47775) (18.286029, 1.46296) (18.331509, 1.447834) (18.376965, 1.432378) (18.422393, 1.416599) (18.467794, 1.400502) (18.513167, 1.38409) (18.558509, 1.367366) (18.603821, 1.350333) (18.649102, 1.332992) (18.694349, 1.315346) (18.739564, 1.297397) (18.784743, 1.279149) (18.829888, 1.260605) (18.874996, 1.241767) (18.920066, 1.222639) (18.965099, 1.203222) (19.010093, 1.18352) (19.055046, 1.163534) (19.099959, 1.143266) (19.144831, 1.122718) (19.18966, 1.101892) (19.234445, 1.08079) (19.279187, 1.059415) (19.323883, 1.037768) (19.368534, 1.015851) (19.413138, 0.993666) (19.457695, 0.971215) (19.502203, 0.948498) (19.546664, 0.925519) (19.591074, 0.902277) (19.635434, 0.878776) (19.679742, 0.855017) (19.723998, 0.831001) (19.768201, 0.806731) (19.812349, 0.782207) (19.856443, 0.75743) (19.900483, 0.732402) (19.935671, 0.712179) (19.962037, 0.696899) (19.979604, 0.686663) (19.988384, 0.681532) knots 0 0 0 0 0 0 0.01428571 0.02857143 0.04285714 0.05714286 0.07142857 0.08571429 0.1 0.11428571 0.12857143 0.14285714 0.15714286 0.17142857 0.18571429 0.2 0.21428571 0.22857143 0.24285714 0.25714286 0.27142857 0.28571429 0.3 0.31428571 0.32857143 0.34285714 0.35714286 0.37142857 0.38571429 0.4 0.41428571 0.42857143 0.44285714 0.45714286 0.47142857 0.48571429 0.5 0.51428571 0.52857143 0.54285714 0.55714286 0.57142857 0.58571429 0.6 0.61428571 0.62857143 0.64285714 0.65714286 0.67142857 0.68571429 0.7 0.71428571 0.72857143 0.74285714 0.75714286 0.77142857 0.78571429 0.8 0.81428571 0.82857143 0.84285714 0.85714286 0.87142857 0.88571429 0.9 0.91428571 0.92857143 0.94285714 0.95714286 0.97142857 0.98571429 1 1 1 1 1 1
  arc A0 (19.988384, -0.681532) -> (19.988384, 0.681532) centre (0, 0) ccw
  line L0 (15.458165, -1.585912) -> (16.82626, -1.72516)
  line L1 (15.458165, 1.585912) -> (16.82626, 1.72516)
  line L2 (15.458165, -1.585912) -> (15.458165, 1.585912)
  point P0 (17.047926, -1.723874)
  point P1 (17.271559, -1.702416)
  point P2 (17.496387, -1.667337)
  point P3 (17.72208, -1.620867)
  point P4 (17.948408, -1.564248)
  point P5 (18.175187, -1.498287)
  point P6 (18.402255, -1.423552)
  point P7 (18.629465, -1.340471)
  point P8 (18.85668, -1.249376)
  point P9 (19.083769, -1.150532)
  point P10 (19.310605, -1.044156)
  point P11 (19.537067, -0.930431)
  point P12 (19.763033, -0.809512)
  point P13 (17.047926, 1.723874)
  point P14 (17.271559, 1.702416)
  point P15 (17.496387, 1.667337)
  point P16 (17.72208, 1.620867)
  point P17 (17.948408, 1.564248)
  point P18 (18.175187, 1.498287)
  point P19 (18.402255, 1.423552)
  point P20 (18.629465, 1.340471)
  point P21 (18.85668, 1.249376)
  point P22 (19.083769, 1.150532)
  point P23 (19.310605, 1.044156)
  point P24 (19.537067, 0.930431)
  point P25 (19.763033, 0.809512)
extrude "Extrude2" add sketch "Sketch2" along normal blind 18 contours S0 S1 A0 L0 L1 L2 picked at (16.370228, -0.528637) in component "Spur Gear (18 teeth)"
fillet "Fillet1" radius 1.1 2 edges at (15.46801, -1.586914, 9) (15.46801, 1.586914, 9) in component "Spur Gear (18 teeth)"
pattern_circular "C-Pattern1" count 18 over 360 about axis through (0, 0, 0) along (0, 0, 1) of "Extrude2", "Fillet1" in component "Spur Gear (18 teeth)"
sketch "Sketch3" plane through (0, 0, 0) normal (0, 0, 1) x (1, 0, 0) in component "Spur Gear (18 teeth)"
  circle A0 centre (0, 0) radius 18 construction
extrude "Extrude3" cut 1 faces at (3.307554, 3.907591, 18) along direction (0, 0, -1) blind 8 in component "Spur Gear (18 teeth)"